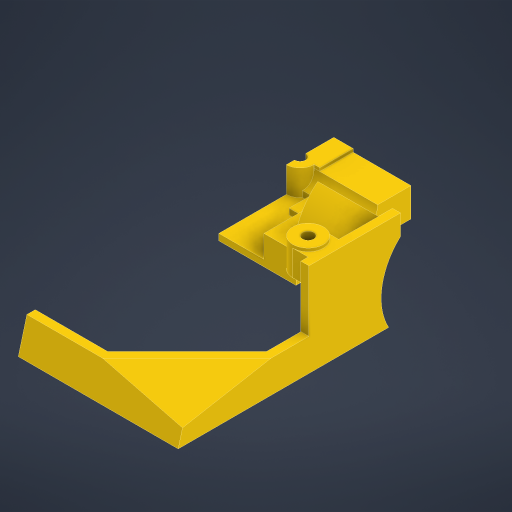
# Autodesk Inventor part: body
Saved by Autodesk Inventor 2024 (Build 280153000, 153)
## iProperties
Created: 2024-01-31
Part Number: body
Material: Všeobecné
Document SubType Name: Modeling
Designer: Simak
Density: 1 g/cm^3
Appearance: Výchozí
Author: Simak
Autodesk Inventor part; units mm, degrees
ref_plane "YZ Plane" through (0, 0, 0) normal (1, 0, 0) x (0, 1, 0)
ref_plane "XZ Plane" through (0, 0, 0) normal (0, 1, 0) x (-1, 0, 0)
ref_plane "XY Plane" through (0, 0, 0) normal (0, 0, 1) x (1, 0, 0)
sketch "Náčrt2" plane through (0, 0, 0) normal (0, 1, 0) x (-1, 0, 0)
  line L0 (0, 49.75) -> (-49.75, 49.75)
  line L1 (-49.75, 49.75) -> (-49.75, -49.75)
  line L2 (-49.75, -49.75) -> (0, -49.75)
  line L3 (-49.75, 49.75) -> (0, 0) construction
  line L4 (0, 0) -> (-49.75, -49.75) construction
  line L5 (-47.25, 49.75) -> (-47.25, -17.75)
  line L6 (-47.25, -17.75) -> (-49.75, -17.75)
  line L7 (0, 49.75) -> (0, -49.75)
  dimension "d0" = 99.5
  dimension "d1" = 67.5
  dimension "d2" = 2.5
  constraints: 16 end point, 5 perpendicular, 2 point on line, 2 vertical, 2 vertical alignment, 1 horizontal
  measures "d0" distance of L0.end L1.end
  measures "d1" distance of L5.start L5.end
  measures "d2" distance of L5.end L6.end
extrude "Vysunutí1" add sketch "Náčrt2" along normal blind 10 contours L5 L6 L1 L0
sketch "Náčrt3" plane through (49.75, 0, 49.75) normal (1, 0, 0) x (0, 0, -1)
  line L0 (67.5, 0) -> (0, 0) projected
  line L1 (67.5, 10) -> (0, 10) projected
  line L2 (0, 0) -> (0, 10) projected
  line L3 (0, 0) -> (0, -5)
  line L4 (0, -5) -> (67.5, -5) construction
  line L5 (67.5, -5) -> (67.5, 0) construction
  line L6 (0, -5) -> (4.0192, 10)
  point P0 (49.75, 0)
  point P1 (1.3397, 0)
  dimension "d8" = 5
  dimension "d9" = 75
  constraints: 8 end point, 2 perpendicular, 1 point on line, 1 vertical
  measures "d8" distance of L4.end L0.start
  measures "d9" angle of L4 L6
extrude "Vysunutí2" cut sketch "Náčrt3" against normal blind 10 contours L0 L2 L1 L6
sketch "Náčrt4" plane through (49.75, 0, -17.75) normal (1, 0, 0) x (0, 0, -1)
  line L0 (0, 10) -> (-63.4808, 10) projected
  line L1 (-60.8926, 10) -> (-63.5721, 0)
  line L2 (0, 0) -> (-66.1603, 0) projected
  line L3 (-63.4808, 10) -> (-66.1603, 0) projected
  point P0 (-17.75, 0)
  dimension "d10" = 2.5
  constraints: 2 end point, 2 point on line, 1 parallel
  measures "d10" distance between parallel lines of L3 L1
extrude "Vysunutí3" add sketch "Náčrt4" against normal up to surface (49.75 mm away)
sketch "Náčrt5" plane through (49.75, 0, -17.75) normal (1, 0, 0) x (0, 0, -1)
  line L0 (-63.4808, 10) -> (0, 10) projected
  line L1 (-25.4808, 10) -> (0, 10)
  line L2 (0, 10) -> (0, 29)
  line L3 (0, 29) -> (-25.4808, 29)
  line L4 (-25.4808, 29) -> (-25.4808, 10)
  point P0 (-17.75, 0)
  dimension "d13" = 38
  dimension "d14" = 19
  constraints: 8 end point, 2 parallel, 1 horizontal, 1 perpendicular, 1 point on line
  measures "d13" distance from line of L4 L0.start
  measures "d14" distance of L3.end L1.start
extrude "Vysunutí4" add sketch "Náčrt5" against normal up to surface (2.5 mm away)
sketch "Náčrt6" plane through (47.25, 0, -17.75) normal (-1, 0, 0) x (0, 0, 1)
  line L0 (63.5721, 0) -> (60.8926, 10) projected
  line L1 (55.5721, 1) -> (63.5721, 1)
  line L2 (63.5721, 1) -> (63.5721, 0)
  line L3 (63.5721, 0) -> (55.5721, 0)
  line L4 (55.5721, 0) -> (55.5721, 1)
  point P0 (17.75, 0)
  dimension "d17" = 1
  dimension "d18" = 8
  constraints: 8 end point, 2 parallel, 1 horizontal, 1 perpendicular
  measures "d17" distance of L3.end L1.start
  measures "d18" distance of L1.start L1.end
extrude "Vysunutí5" add sketch "Náčrt6" along normal up to surface (47.25 mm away)
sketch "Náčrt7" plane through (47.25, 0, -17.75) normal (-1, 0, 0) x (0, 0, 1)
  line L0 (60.8926, 10) -> (63.3041, 1) projected
  line L1 (62.7682, 3) -> (63.3041, 3)
  line L2 (63.3041, 3) -> (63.3041, 1)
  line L3 (63.3041, 1) -> (62.7682, 1)
  line L4 (62.7682, 1) -> (62.7682, 3)
  point P0 (17.75, 0)
  dimension "d21" = 2
  constraints: 8 end point, 2 parallel, 1 horizontal, 1 perpendicular, 1 point on line
  measures "d21" distance of L3.end L1.start
extrude "Vysunutí6" cut sketch "Náčrt7" along normal up to surface (47.25 mm away) contours L1 L2 L0
sketch "Náčrt8" plane through (0, 10, 0) normal (0, 1, 0) x (1, 0, 0)
  line L0 (49.75, -45.7308) -> (49.75, -7.7308) projected
  point P0 (0, 0)
  point P1 (23.5355, -45.7308)
  point P2 (49.75, -19.5163)
  dimension "d24" = 26.2145
  dimension "d25" = 26.2145
  constraints: 1 horizontal alignment, 1 point on line, 1 vertical alignment
  measures "d24" distance from line of L0 point (23.536, -45.731)
  measures "d25" distance of L0.start point (49.75, -19.516)
sketch "Náčrt9" plane through (49.75, 0, 48.4103) normal (1, 0, 0) x (0, 0, -1)
  line L0 (1.3397, 5) -> (0, 0) construction
  line L1 (2.6795, 10) -> (5.2677, 10) projected
  line L2 (1.3397, 5) -> (2.6795, 10) construction
  point P0 (48.4103, 0)
  constraints: 4 end point, 2 collinear
ref_plane "Pracovní rovina1" through (23.5355, 10, 45.7308) normal (-0.1757652, -0.9686141, -0.1757652) x (0.7071068, 0, -0.7071068)
sketch "Náčrt10" plane through (23.5355, 10, 45.7308) normal (-0.1757652, -0.9686141, -0.1757652) x (0.7071068, 0, -0.7071068)
  line L0 (18.5364, 17.9546) -> (-16.6421, -16.1198) projected
  line L1 (0, 0) -> (17.5891, 20.1151)
  line L2 (18.5364, 17.9546) -> (16.6417, 22.2756) projected
  line L3 (17.5891, 20.1151) -> (37.0729, 0)
  line L4 (0, 0) -> (37.0729, 0)
  point P0 (15.6944, -44.9557)
  point P1 (37.0729, 0)
  constraints: 6 end point, 1 coincident, 1 horizontal, 1 midpoint
extrude "Vysunutí7" cut sketch "Náčrt10" against normal blind 10
sketch "Náčrt11" plane through (23.5355, 10, 45.7308) normal (0.1757652, 0.9686141, 0.1757652) x (0.6849136, -0.2485695, 0.6849136)
  line L0 (0, 3.6603) -> (16.2108, 17.8353) projected
  line L1 (0, 0) -> (0, 3.6603) projected
  line L2 (20.1151, 17.5891) -> (0, 0) projected
  line L3 (0, 37.0729) -> (20.1151, 17.5891) projected
  line L4 (0, 33.5373) -> (0, 37.0729) projected
  line L5 (16.2108, 17.8353) -> (0, 33.5373) projected
  line L6 (0, 3.6603) -> (0, 33.5373)
  point P0 (-44.9557, 15.6944)
  constraints: 2 end point, 1 vertical
extrude "Vysunutí8" add sketch "Náčrt11" against normal blind 1.5
sketch "Náčrt13" plane through (23.2719, 8.5471, 45.4671) normal (-0.1757652, -0.9686141, -0.1757652) x (0.7071068, 0, -0.7071068)
  line L0 (17.5269, 16.9141) -> (33.9102, 0) projected
  line L1 (2.7368, 0) -> (17.5269, 16.9141) projected
  line L2 (2.7368, 0) -> (33.9102, 0) projected
  line L3 (33.9102, 0) -> (36.2562, -2.422)
  line L4 (43.6387, -9.7844) -> (33.5373, 0) projected
  line L5 (36.2562, -2.422) -> (0.619, -2.422)
  line L6 (0.619, -2.422) -> (2.7368, 0)
  point P0 (15.6944, -44.9557)
  point P1 (39.5718, -5.8451)
  point P2 (2.7368, 0)
  point P3 (36.0378, -2.422)
  dimension "d30" = 2.422
  constraints: 6 end point, 2 collinear, 2 point on line, 1 horizontal
  measures "d30" distance between parallel lines of L2 L5
extrude "Vysunutí9" add sketch "Náčrt13" against normal up to surface contours L3 L5 L4 L2 | L2 L4 L5 L6 surface through (48.5, 10, 16) normal (0, 1, 0)
sketch "Náčrt14" plane through (0, 0, 0) normal (0, -1, 0) x (1, 0, 0)
  line L0 (47.25, 37.8221) -> (0, 37.8221) projected
  line L1 (44.25, 37.8221) -> (36.75, 37.8221)
  line L2 (36.75, 37.8221) -> (36.75, 41.8041)
  line L3 (44.25, 41.8041) -> (44.25, 37.8221)
  line L4 (49.75, 48.4103) -> (49.75, -17.75) projected
  line L5 (49.75, 48.4103) -> (0, 48.4103) projected
  arc A0 (44.25, 41.8041) -> (36.75, 41.8041) centre (40.5, 41.8041) ccw
  line L6 (47.25, 45.5541) -> (0, 45.5541) projected
  line L7 (47.25, 45.5541) -> (0, 45.5541) projected
  point P0 (0, 0)
  point P1 (36.75, 37.8221)
  point P2 (40.5, 45.5541)
  dimension "d33" = 5.5
  dimension "d35" = 7.5
  constraints: 6 end point, 3 point on circle, 2 point on line, 2 tangent, 1 centre point, 1 horizontal, 1 parallel, 1 perpendicular
  measures "d33" distance between parallel lines of L4 L3
  measures "d35" distance of L2.end L3.start
extrude "Vysunutí10" cut sketch "Náčrt14" against normal up to surface (1 mm away)
sketch "Náčrt15" plane through (47.25, 0, -17.75) normal (-1, 0, 0) x (0, 0, 1)
  circle A0 centre (-15.5, 9) radius 18.5
  line L0 (0, 0) -> (0, 29) projected
  line L1 (0, 0) -> (55.5721, 0) projected
  circle A1 centre (-15.5, 9) radius 20
  line L2 (-3, 24.6125) -> (-3, 22.6382)
  point P0 (17.75, 0)
  point P1 (0, 21.6392)
  point P2 (0, 19.0995)
  point P3 (0.6632, 0)
  point P4 (2.3606, 0)
  point P5 (0, 0.876)
  dimension "d39" = 37
  dimension "d41" = 1.5
  dimension "d38" = 15.5
  dimension "d44" = 9
  dimension "d47" = 6
  constraints: 2 end point, 1 vertical, 6 other
  measures "d38" distance from line of L0 point (-15.5, 9)
  measures "d44" distance from line of L1 point (-15.5, 9)
extrude "Vysunutí11" cut sketch "Náčrt15" against normal up to surface (2.5 mm away) contours A0 L1 L0 | L0 L1 A0
extrude "Vysunutí12" add sketch "Náčrt15" along normal blind 25 contours A0 L0 A1 L1 | A0 L2 A1 L0
sketch "Náčrt16" plane through (49.75, 29, 7.7308) normal (0, 1, 0) x (1, 0, 0)
  line L0 (-2.5, 28.4808) -> (-2.5, 25.4808) projected
  line L1 (0, 25.4808) -> (-2.5, 25.4808) projected
  line L2 (-2.5, 25.4808) -> (0, 25.4808)
  line L3 (0, 25.4808) -> (0, 28.4808)
  line L4 (0, 28.4808) -> (-2.5, 28.4808)
  line L5 (-2.5, 28.4808) -> (-2.5, 25.4808)
  point P0 (-49.75, 7.7308)
  point P1 (-2.5, 23.1202)
  constraints: 8 end point, 4 parallel, 1 horizontal, 1 perpendicular
extrude "Vysunutí13" add sketch "Náčrt16" against normal up to surface round surface about axis through (47.25, 9, -33.25) along (1, 0, 0) radius 18.5 far side no
sketch "Náčrt18" plane through (47.25, 29, 7.7308) normal (0, 1, 0) x (1, 0, 0)
  circle A0 centre (-4.75, 7) radius 4.75
  line L0 (0, 28.4808) -> (0, 0) projected
  line L1 (2.5, 0) -> (0, 0) projected
  line L2 (2.5, 28.4808) -> (2.5, 0) projected
  line L3 (2.5, 28.4808) -> (0, 28.4808) projected
  line L4 (-4.75, 2.25) -> (0, 2.25)
  line L5 (-4.75, 11.75) -> (0, 11.75)
  circle A1 centre (-4.75, 7) radius 1.75
  point P0 (-47.25, 7.7308)
  dimension "d51" = 3.5
  dimension "d52" = 3
  dimension "d53" = 4.75
  dimension "d54" = 7
  constraints: 4 end point, 2 centre point, 2 point on circle, 2 point on line, 1 coincident, 1 horizontal, 1 parallel, 1 perpendicular, 1 tangent
  measures "d51" diameter of A1
  measures "d52" radial gap between concentric circles of A0 A1
  measures "d53" distance from line of L0 A0.centre
  measures "d54" distance from line of L1 A0.centre
extrude "Vysunutí14" add sketch "Náčrt18" against normal blind 8 contours A0 | L0 L4 A0 | A0 L5 L0
extrude "Vysunutí15" add sketch "Náčrt18" along normal blind 1 contours A0
sketch "Náčrt20" plane through (0, 0, 0) normal (0, -1, 0) x (1, 0, 0)
  line L0 (0, -14) -> (24, -14)
  line L1 (24, -14) -> (24, -49.75)
  line L2 (24, -49.75) -> (0, -49.75)
  line L3 (0, -49.75) -> (0, -14)
  line L4 (22.25, -20.75) -> (49.75, -20.75) projected
  point P0 (0, 0)
  dimension "d63" = 29
  dimension "d82" = 14
  constraints: 8 end point, 2 parallel, 1 horizontal, 1 perpendicular, 1 vertical alignment
  measures "d63" distance between parallel lines of L4 L2
  measures "d82" distance from line of point (0, 0) L0
extrude "Vysunutí16" add sketch "Náčrt20" against normal blind 9
sketch "Náčrt21" plane through (24, 0, -17.0868) normal (1, 0, 0) x (0, 0, -1)
  line L0 (12.7467, 3.9) -> (19.5797, 3.9)
  line L1 (-2.3368, 9) -> (32.6632, 9) projected
  arc A0 (19.5797, 3.9) -> (22.3018, 9) centre (16.1632, 9) ccw
  arc A1 (10.0246, 9) -> (12.7467, 3.9) centre (16.1632, 9) ccw
  line L2 (32.6632, 0) -> (32.6632, 9) projected
  point P0 (-17.0868, 0)
  point P1 (-1.6973, 9)
  dimension "d66" = 5.1
  dimension "d67" = 16.5
  dimension "d68" = 6.833
  constraints: 4 point on circle, 2 centre point, 2 end point, 2 line through centre, 2 point on line, 1 coincident, 1 concentric, 1 horizontal
  measures "d66" distance between parallel lines of L0 L1
  measures "d67" distance from line of L2 A0.centre
  measures "d68" distance of L0.start L0.end
extrude "Vysunutí17" cut sketch "Náčrt21" against normal up to next
sketch "Náčrt23" plane through (24, 0, -49.75) normal (0, 0, -1) x (-1, 0, 0)
  line L0 (0, 3.9) -> (24, 3.9) projected
  line L1 (0, 3.9) -> (24, 3.9) projected
  line L2 (18, 3.9) -> (18, 9)
  line L3 (24, 0) -> (0, 0) projected
  line L4 (24, 0) -> (24, 9) projected
  line L5 (0, 9) -> (24, 9) projected
  line L6 (0, 0) -> (0, 9) projected
  point P0 (24, 0)
  dimension "d73" = 18
  constraints: 2 end point, 2 point on line, 1 perpendicular
  measures "d73" distance between parallel lines of L6 L2
extrude "Vysunutí19" cut sketch "Náčrt23" against normal up to surface (35.75 mm away) contours L2 L5 L4 L0
sketch "Náčrt24" plane through (0, 9, 0) normal (0, 1, 0) x (1, 0, 0)
  line L0 (22.25, 14) -> (22.25, 20.75) projected
  line L1 (47.25, 15.3894) -> (24, 15.3894) projected
  line L2 (47.25, 20.75) -> (47.25, 15.3894) projected
  line L3 (47.25, 20.75) -> (22.25, 20.75) projected
  line L4 (6, 27.1114) -> (6, 14) projected
  line L5 (24, 14.75) -> (22.25, 14.75) projected
  line L6 (24, 27.1114) -> (6, 27.1114) projected
  line L7 (24, 29.8335) -> (6, 29.8335) projected
  line L8 (24, 36.6665) -> (24, 29.8335) projected
  line L9 (24, 36.6665) -> (6, 36.6665) projected
  line L10 (6, 49.75) -> (6, 36.6665) projected
  line L11 (0, 49.75) -> (6, 49.75) projected
  line L12 (0, 14) -> (0, 49.75) projected
  line L13 (6, 29.8335) -> (6, 14) projected
  line L14 (47.25, 13.25) -> (22.25, 13.25) projected
  line L15 (22.25, 20.75) -> (22.25, 13.25) projected
  line L16 (24, 14.75) -> (24, 13.25)
  line L17 (6, 29.8335) -> (0, 29.8335)
  line L18 (6, 36.6665) -> (6, 29.8335)
  line L19 (6, 36.6665) -> (0, 36.6665)
  line L20 (22.25, 14) -> (24, 14) projected
  line L21 (24, 14) -> (24, 15.3894) projected
  line L22 (6, 14) -> (0, 14) projected
  line L23 (22.25, 14.75) -> (22.25, 14) projected
  line L24 (24, 14.75) -> (24, 27.1114) projected
  line L25 (6, 49.75) -> (6, 39.3886) projected
  line L26 (6, 39.3886) -> (24, 39.3886) projected
  line L27 (24, 39.3886) -> (24, 49.75) projected
  line L28 (24, 49.75) -> (6, 49.75) projected
  line L29 (6, 14) -> (22.25, 14) projected
  line L30 (14, 29.8335) -> (14, 14)
  point P0 (0, 0)
  point P1 (22.25, 15.3894)
  point P2 (22.25, 15.3894)
  point P3 (22.25, 13.25)
  point P4 (24, 20.75)
  dimension "d84" = 10
  constraints: 10 end point, 5 perpendicular, 5 point on line
  measures "d84" distance between parallel lines of L24 L30
extrude "Vysunutí20" cut sketch "Náčrt24" along normal up to next contours L20 L16 L14 L15 | L0 L5 L16 L20 | L0 L3 L24 L21 L5
extrude "Vysunutí21" cut sketch "Náčrt24" against normal blind 7 contours L29 L4 L6 L30 | L22 L12 L17 L13 L4 | L6 L13 L7 L30 | L17 L12 L19 L18
sketch "Náčrt25" plane through (0, 3.9, -49.75) normal (0, 1, 0) x (1, 0, 0)
  line L0 (0, -13.0835) -> (6, -13.0835) projected
  line L1 (6, 0) -> (6, -13.0835) projected
  line L2 (0, 0) -> (6, 0) projected
  line L3 (0, -13.0835) -> (0, 0) projected
  line L4 (6, 0) -> (6, -10.3614) projected
  line L5 (6, -10.3614) -> (24, -10.3614) projected
  line L6 (24, -10.3614) -> (24, 0) projected
  line L7 (24, 0) -> (6, 0) projected
  line L8 (6, -10.3614) -> (0, -10.3614)
  point P0 (0, -49.75)
  constraints: 2 end point, 1 perpendicular, 1 point on line
extrude "Vysunutí22" add sketch "Náčrt25" along normal blind 6.1 contours L3 L8 L1 L0 | L3 L2 L1 L8
sketch "Náčrt26" plane through (0, 10, -49.75) normal (0, 1, 0) x (1, 0, 0)
  circle A0 centre (0, -10.4808) radius 1.75
  line L0 (49.75, -57.4808) -> (47.25, -57.4808) projected
  circle A1 centre (0, -10.4808) radius 4.25
  line L1 (6, 0) -> (6, -10.3614) projected
  line L2 (6, -10.3614) -> (24, -10.3614) projected
  line L3 (24, -10.3614) -> (24, 0) projected
  line L4 (24, 0) -> (6, 0) projected
  line L5 (0, 0) -> (0, -13.0835) projected
  line L6 (0, -13.0835) -> (6, -13.0835) projected
  line L7 (6, -13.0835) -> (6, 0) projected
  line L8 (6, 0) -> (0, 0) projected
  line L9 (6, -10.3614) -> (4.25, -10.3614)
  line L10 (4.25, -10.3614) -> (4.25, -10.4808)
  line L11 (0, -13.0835) -> (6, -13.0835) projected
  line L12 (0, -35.75) -> (0, -13.0835) projected
  line L13 (14, -35.75) -> (0, -35.75) projected
  line L14 (14, -19.9165) -> (14, -35.75) projected
  line L15 (6, -19.9165) -> (14, -19.9165) projected
  line L16 (6, -13.0835) -> (6, -19.9165) projected
  point P0 (0, -49.75)
  point P1 (0, -6.2308)
  point P2 (0, -8.7308)
  point P3 (0, -12.2308)
  point P4 (0, -14.7308)
  point P5 (3.3598, -13.0835)
  dimension "d87" = 47
  dimension "d88" = 2.5
  dimension "d89" = 3.5
  constraints: 4 end point, 1 centre point, 1 horizontal, 1 perpendicular, 1 vertical, 1 vertical alignment, 3 other
  measures "d87" distance from line of L0 A0.centre
  measures "d89" diameter of A0
extrude "Vysunutí23" add sketch "Náčrt26" against normal up to next contours A0 L5 A1 L6 | L6 A1 L12
extrude "Vysunutí24" cut sketch "Náčrt26" against normal up to next contours A0 L5 picked at (0.3637, -10.0247)
extrude "Vysunutí25" cut sketch "Náčrt26" against normal up to surface (8 mm away) contours L9 L7 L6 A1
sketch "Náčrt27" plane through (6, 2, -29.8335) normal (-1, 0, 0) x (0, 0, 1)
  line L0 (-6.833, 1.9) -> (0, 1.9) projected
  arc A0 (-9.5551, 7) -> (-6.833, 1.9) centre (-3.4165, 7) ccw projected
  line L1 (-9.5551, 7) -> (-9.5551, 0) projected
  line L2 (-9.5551, 0) -> (0, 0) projected
  line L3 (0, 1.9) -> (0, 0) projected
  line L4 (-6.833, 1.9) -> (-3.9968, 0)
  line L5 (-6.833, 1.9) -> (-6.833, 0)
  point P0 (29.8335, -2)
  constraints: 4 end point, 2 point on line, 1 perpendicular, 1 tangent
extrude "Vysunutí26" add sketch "Náčrt27" along normal up to next contours L5 L2 L1 A0
sketch "Náčrt28" plane through (0, 0, 0) normal (0, -1, 0) x (1, 0, 0)
  arc A0 (0, -41.0192) -> (0, -37.5192) centre (0, -39.2692) ccw projected
  line L0 (0, -14) -> (0, -35.0192) projected
  line L1 (0, -35.9783) -> (2.85, -37.6238)
  line L2 (2.85, -37.6238) -> (2.85, -40.9147)
  line L3 (2.85, -40.9147) -> (0, -42.5601)
  line L4 (0, -42.5601) -> (-2.85, -40.9147)
  line L5 (-2.85, -40.9147) -> (-2.85, -37.6238)
  line L6 (-2.85, -37.6238) -> (0, -35.9783)
  arc A1 (0, -41.0192) -> (0, -37.5192) centre (0, -39.2692) ccw projected
  line L7 (0, -41.0192) -> (0, -49.75) projected
  line L8 (0, -49.75) -> (24, -49.75) projected
  line L9 (24, -49.75) -> (24, -17.0868) projected
  line L10 (24, -17.0868) -> (49.75, -17.0868) projected
  line L11 (49.75, 48.4103) -> (49.75, -17.0868) projected
  line L12 (49.75, 48.4103) -> (0, 48.4103) projected
  line L13 (0, 37.8221) -> (0, 48.4103) projected
  line L14 (36.75, 37.8221) -> (0, 37.8221) projected
  line L15 (36.75, 37.8221) -> (36.75, 41.8041) projected
  arc A2 (44.25, 41.8041) -> (36.75, 41.8041) centre (40.5, 41.8041) ccw projected
  line L16 (44.25, 41.8041) -> (44.25, 37.8221) projected
  line L17 (47.25, 37.8221) -> (44.25, 37.8221) projected
  line L18 (47.25, -15.3894) -> (47.25, 37.8221) projected
  line L19 (47.25, -15.3894) -> (24, -15.3894) projected
  line L20 (24, -15.3894) -> (24, -14) projected
  line L21 (24, -14) -> (0, -14) projected
  line L22 (0, -14) -> (0, -37.5192) projected
  point P0 (0, 0)
  point P1 (0, -37.5192)
  point P2 (0, -41.0192)
  point P3 (0, -42.5601)
  dimension "d98" = 5.7
  constraints: 12 end point, 1 coincident, 1 point on line, 13 other
  measures "d98" distance between parallel lines of L4 L1
extrude "Vysunutí27" cut sketch "Náčrt28" against normal blind 6 contours A0 L22 L1 L2 L3 L7
chamfer "Zkosení1" distance 0.7 angle 45 1 edges at (1.75, 6, -39.2692)
